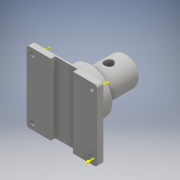
# Autodesk Inventor part: adaptor
Saved by Autodesk Inventor 2016 (Build 200138000, 138)
## iProperties
Created: 2018-10-09
Part Number: adaptor
Material: Generic
Document SubType Name: Modeling
Designer: andrew
Density: 1 g/cm^3
Appearance: Default
Author: andrew
Autodesk Inventor part; units mm, degrees
ref_plane "YZ Plane" through (0, 0, 0) normal (1, 0, 0) x (0, 1, 0)
ref_plane "XZ Plane" through (0, 0, 0) normal (0, 1, 0) x (-1, 0, 0)
ref_plane "XY Plane" through (0, 0, 0) normal (0, 0, 1) x (1, 0, 0)
sketch "Sketch1" plane through (0, 0, 0) normal (0, 1, 0) x (-1, 0, 0)
  line L0 (24, 24) -> (-24, 24)
  line L1 (-24, 24) -> (-24, -24)
  line L2 (-24, -24) -> (24, -24)
  line L3 (24, -24) -> (24, 24)
  line L4 (24, 24) -> (-24, -24) construction
  line L5 (-24, 24) -> (24, -24) construction
  point P0 (0, 0)
  dimension "d0" = 48
  dimension "d1" = 48
  constraints: 12 end point, 2 midpoint, 2 parallel, 1 horizontal, 1 perpendicular
  measures "d0" distance of L2.end L1.end
  measures "d1" distance of L1.end L0.end
extrude "Extrusion1" add sketch "Sketch1" along normal blind 4
sketch "Sketch2" plane through (0, 4, 0) normal (0, 1, 0) x (1, 0, 0)
  circle A0 centre (0, 0) radius 15
  dimension "d4" = 30
  constraints: 1 centre point, 1 coincident
  measures "d4" diameter of A0
extrude "Extrusion2" add sketch "Sketch2" along normal blind 15
fillet "Fillet1" radius 7 1 edges at (-15, 4, 0)
sketch "Sketch4" plane through (0, 4, 0) normal (0, 1, 0) x (1, 0, 0)
  line L0 (20, 20) -> (-20, 20) construction
  line L1 (-20, 20) -> (-20, -20) construction
  line L2 (-20, -20) -> (20, -20) construction
  line L3 (20, -20) -> (20, 20) construction
  line L4 (20, 20) -> (-20, -20) construction
  line L5 (-20, 20) -> (20, -20) construction
  point P0 (0, 0)
  dimension "d11" = 40
  dimension "d12" = 40
  constraints: 12 end point, 2 midpoint, 2 parallel, 1 horizontal, 1 perpendicular
  measures "d11" distance of L2.end L1.end
  measures "d12" distance of L1.end L0.end
hole "Hole1" at (-20, 4, 20) at (-20, 4, -20) at (20, 4, 20) at (20, 4, -20) direction (0, -1, 0) diameter 3 end through all
fillet "Fillet2" radius 2 4 edges at (24, 2, 24) (-24, 2, 24) (24, 2, -24) (-24, 2, -24)
sketch "Sketch5" plane through (22, 0, -24) normal (0, 0, -1) x (-1, 0, 0)
  line L0 (14.5, -3) -> (29.5, -3)
  line L1 (29.5, -3) -> (29.5, 3)
  line L2 (29.5, 3) -> (14.5, 3)
  line L3 (14.5, 3) -> (14.5, -3)
  line L4 (14.5, -3) -> (29.5, 3) construction
  line L5 (29.5, -3) -> (14.5, 3) construction
  point P0 (22, 0)
  dimension "d21" = 15
  dimension "d22" = 6
  constraints: 12 end point, 2 midpoint, 2 parallel, 1 horizontal, 1 perpendicular
  measures "d21" distance of L2.end L1.end
  measures "d22" distance of L1.end L0.end
extrude "Extrusion4" cut sketch "Sketch5" against normal blind 80
sketch "Sketch6" plane through (0, 19, 0) normal (0, 1, 0) x (1, 0, 0)
  circle A0 centre (0, 0) radius 9.75
  dimension "d25" = 19.5
  constraints: 1 centre point, 1 coincident
  measures "d25" diameter of A0
extrude "Extrusion5" add sketch "Sketch6" along normal blind 25
fillet "Fillet3" radius 3 1 edges at (-9.75, 44, 0)
sketch "Sketch7" plane through (-22, 4, 24) normal (0, 0, 1) x (1, 0, 0)
  line L0 (22, -4) -> (22, 27.5) construction
  dimension "d29" = 31.5
  constraints: 2 end point, 1 vertical
  measures "d29" distance of L0.start L0.end
hole "Hole2" at (0, 31.5, 24) direction (0, 0, -1) diameter 6 end through all
body "Solid1"
